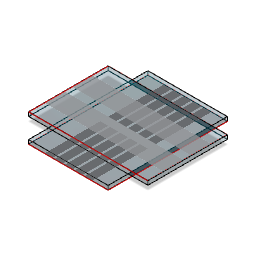
Assmbly (Autodesk Fusion 360 archive; units mm, degrees)
design "TCA Test Structure"
Autodesk Fusion 360 part; units mm, degrees
sketch "Sketch1" plane through (0, 0, 0) normal (0, 1, 0) x (1, 0, 0)
  line L0 (10, -15) -> (-10, -15)
  line L1 (-10, -15) -> (-10, 15)
  line L2 (-10, 15) -> (10, 15)
  line L3 (10, 15) -> (10, -15)
  line L4 (10, -15) -> (-10, 15) construction
  line L5 (-10, -15) -> (10, 15) construction
  dimension "d1" = 20
  dimension "d2" = 30
  constraint perpendicular L0 L1
  constraint parallel L0 L2
  constraint parallel L1 L3
  constraint horizontal L0
  constraint coincident L4 origin
  constraint coincident L5 origin
  measures "d1" distance of L1.end L2.end
  measures "d2" distance of L0.end L1.end
extrude "Extrude1" add sketch "Sketch1" along normal blind 1
sketch "Sketch2" plane through (0, 1, 0) normal (0, 1, 0) x (-1, 0, 0)
  line L0 (-10, -15) -> (10, -15)
  line L1 (10, -15) -> (10, 15)
  line L2 (10, 15) -> (-10, 15)
  line L3 (-10, 15) -> (-10, -15)
  line L4 (-10, 10) -> (10, 10)
  line L5 (10, 10) -> (10, -10)
  line L6 (10, -10) -> (-10, -10)
  line L7 (-10, -10) -> (-10, 10)
  line L8 (-10, 10) -> (10, -10) construction
  line L9 (10, 10) -> (-10, -10) construction
  dimension "d5" = 20
  constraint perpendicular L4 L5
  constraint parallel L4 L6
  constraint parallel L5 L7
  constraint horizontal L4
  constraint coincident L3 L4.start
  constraint coincident L8 origin
  constraint coincident L9 origin
  measures "d5" distance of L4.end L5.end
extrude "Extrude2" add sketch "Sketch2" along normal blind 0.04 contours L1 L3 L4 L5 L6 L7
sketch "Sketch3" plane through (0, 1.04, 0) normal (0, 1, 0) x (-1, 0, 0)
  line L0 (-10, -10) -> (10, -10)
  line L1 (10, -10) -> (10, 10)
  line L2 (10, 10) -> (-10, 10)
  line L3 (-10, 10) -> (-10, -10)
  line L4 (-15, 10) -> (15, 10)
  line L5 (15, 10) -> (15, -10)
  line L6 (15, -10) -> (-15, -10)
  line L7 (-15, -10) -> (-15, 10)
  line L8 (-15, 10) -> (15, -10) construction
  line L9 (15, 10) -> (-15, -10) construction
  dimension "d8" = 30
  dimension "d9" = 20
  constraint perpendicular L4 L5
  constraint parallel L4 L6
  constraint parallel L5 L7
  constraint horizontal L4
  constraint coincident L8 origin
  constraint coincident L9 origin
  measures "d8" distance of L5.end L6.end
  measures "d9" distance of L4.end L5.end
extrude "Extrude3" add sketch "Sketch3" along normal blind 1
